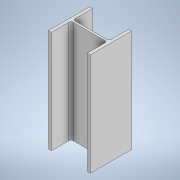
# Autodesk Inventor part: Pierwszy projekt
Saved by Autodesk Inventor 2021 (Build 250183000, 183)
## iProperties
Created: 2020-04-11
Part Number: Pierwszy projekt
Material: Ogólny
Document SubType Name: Modeling
Designer: dyrag
Density: 1 g/cm^3
Appearance: Domyślna
Author: dyrag
Autodesk Inventor part; units mm, degrees
ref_plane "YZ Plane" through (0, 0, 0) normal (1, 0, 0) x (0, 1, 0)
ref_plane "XZ Plane" through (0, 0, 0) normal (0, 1, 0) x (-1, 0, 0)
ref_plane "XY Plane" through (0, 0, 0) normal (0, 0, 1) x (1, 0, 0)
sketch "Szkic1" plane through (0, 0, 0) normal (0, 1, 0) x (-1, 0, 0)
  line L0 (0, 0) -> (0, -200)
  line L1 (0, -200) -> (15, -200)
  line L2 (15, -200) -> (15, -105)
  line L3 (15, -105) -> (190, -105)
  line L4 (190, -105) -> (190, -200)
  line L5 (190, -200) -> (205, -200)
  line L6 (205, -200) -> (205, 0)
  line L7 (205, 0) -> (190, 0)
  line L8 (190, 0) -> (190, -95)
  line L9 (190, -95) -> (15, -95)
  line L10 (15, -95) -> (15, 0)
  line L11 (15, 0) -> (0, 0)
  line L12 (15, 0) -> (0, 0)
  dimension "d0" = 200
  dimension "d1" = 15
  dimension "d2" = 95
  dimension "d3" = 175
  dimension "d4" = 15
  dimension "d5" = 95
  constraints: 26 end point, 7 perpendicular, 7 point on line, 1 collinear, 1 horizontal, 1 vertical
  measures "d0" distance of L0.start L0.end
  measures "d1" distance of L0.end L1.end
  measures "d2" distance of L1.end L2.end
  measures "d3" distance of L2.end L3.end
  measures "d4" distance of L4.end L5.end
  measures "d5" distance of L7.end L8.end
extrude "Wyciągnięcie proste1" add sketch "Szkic1" along normal mid plane 500
fillet "Zaokrąglenie2" radius 10 4 edges at (-190, 0, -105) (-15, 0, -105) (-15, 0, -95) (-190, 0, -95)
